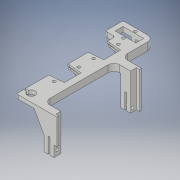
# Autodesk Inventor part: stand2
Saved by Autodesk Inventor 2019 (Build 230136000, 136)
## iProperties
Created: 2019-09-12
Part Number: stand2
Material: Generic
Document SubType Name: Modeling
Designer: James
Density: 1 g/cm^3
Appearance: Default
Author: James
Autodesk Inventor part; units mm, degrees
ref_plane "YZ Plane" through (0, 0, 0) normal (1, 0, 0) x (0, 1, 0)
ref_plane "XZ Plane" through (0, 0, 0) normal (0, 1, 0) x (-1, 0, 0)
ref_plane "XY Plane" through (0, 0, 0) normal (0, 0, 1) x (1, 0, 0)
sketch "Sketch1" plane through (0, 0, 0) normal (0, 1, 0) x (-1, 0, 0)
  line L0 (-9.5, 50) -> (-9.5, -50)
  line L1 (-9.5, -50) -> (9.5, -50)
  line L2 (9.5, 50) -> (9.5, -50)
  line L3 (-9.5, 50) -> (9.5, 50)
  line L4 (9.5, -24) -> (-3, -24)
  line L5 (-3, -24) -> (-3, -41)
  line L6 (-3, -41) -> (9.5, -41)
  line L7 (9.5, -41) -> (9.5, -24)
  circle A0 centre (3.25, -45) radius 1.5
  circle A1 centre (3.25, -20) radius 1.5
  line L8 (9.5, 16) -> (-3, 16)
  line L9 (-3, 16) -> (-3, -1)
  line L10 (-3, -1) -> (9.5, -1)
  circle A2 centre (3.25, -5) radius 1.5
  circle A3 centre (3.25, 20) radius 1.5
  arc A4 (8.4291, 42.75) -> (8.2997, 40.75) centre (4.5, 42) ccw
  line L11 (6.5529, 38) -> (0.8469, 38)
  line L12 (9.5, 42.75) -> (8.4291, 42.75)
  line L13 (8.2997, 40.75) -> (9.5, 40.75)
  point P0 (0, 0)
  point P1 (9.5, 0)
  point P2 (-9.5, 0)
  point P3 (-3, -32.5)
  point P4 (3.25, -24)
  point P5 (0, -50)
  point P6 (-3, 7.5)
  point P7 (3.25, 16)
  dimension "d3" = 17
  dimension "d4" = 12.5
  dimension "d5" = 12.5
  dimension "d6" = 12.5
  dimension "d7" = 100
  dimension "d8" = 19
  dimension "d9" = 17
  dimension "d10" = 12.5
  dimension "d11" = 12.5
  dimension "d12" = 12.5
  dimension "d13" = 40
  dimension "d14" = 3
  dimension "d15" = 17.5
  dimension "d16" = 8
  dimension "d18" = 5
  dimension "d19" = 2
  dimension "d20" = 0.75
  dimension "d68" = 8
  constraints: 28 end point, 7 midpoint, 7 perpendicular, 5 centre point, 5 point on line, 5 vertical alignment, 4 horizontal, 3 equal radius, 3 parallel, 2 horizontal alignment, 2 point on circle, 1 tangent
  measures "d3" distance of L4.end L5.end
  measures "d4" distance of L4.start L4.end
  measures "d5" vertical distance of A1.centre point (-3, -32.5)
  measures "d6" vertical distance of A0.centre point (-3, -32.5)
  measures "d7" distance of L2.start L1.end
  measures "d8" distance of L0.start L2.start
  measures "d9" distance of L8.end L9.end
  measures "d10" distance of L8.start L8.end
  measures "d11" vertical distance of A3.centre point (-3, 7.5)
  measures "d12" vertical distance of A2.centre point (-3, 7.5)
  measures "d13" distance of point (-3, -32.5) point (-3, 7.5)
  measures "d14" diameter of A3
  measures "d15" distance from line of L1 point (-3, -32.5)
  measures "d16" diameter of A4
  measures "d18" distance from line of L2 A4.centre
  measures "d19" distance between parallel lines of L13 L12
  measures "d20" vertical distance of A4.centre L12.start
  measures "d68" distance from line of L3 A4.centre
extrude "Extrusion1" add sketch "Sketch1" along normal blind 3 contours L3 L2 L12 A4 L13 L8 L9 L10 L4 L5 L6 L1 L0
sketch "Sketch2" plane through (-9.5, 0, 16) normal (-1, 0, 0) x (0, 0, 1)
  line L0 (-64.2, 0.85) -> (-64.2, 2.15)
  line L1 (7.2, 2.15) -> (7.2, 0.85)
  line L2 (-66, 0) -> (-66, 3) projected
  line L3 (-66, 3) -> (-57, 3) projected
  line L4 (-24.2, 0.85) -> (-24.2, 2.15)
  line L5 (-32.8, 0.85) -> (-32.8, 2.15)
  line L6 (-64.2, 2.15) -> (-32.8, 2.15)
  line L7 (-24.2, 2.15) -> (7.2, 2.15)
  line L8 (7.2, 0.85) -> (-24.2, 0.85)
  line L9 (-32.8, 0.85) -> (-64.2, 0.85)
  point P0 (-16, 0)
  point P1 (-24.2, 1.5)
  point P2 (-32.8, 1.5)
  point P3 (-64.2, 1.5)
  point P4 (-66, 1.5)
  dimension "d23" = 1.3
  dimension "d57" = 1.8
  dimension "d58" = 8.6
  dimension "d59" = 31.4
  dimension "d60" = 31.4
  dimension "d61" = 1.3
  constraints: 16 end point, 5 parallel, 4 midpoint, 4 perpendicular, 2 horizontal, 2 horizontal alignment
  measures "d23" distance of L1.end L1.start
  measures "d57" distance between parallel lines of L2 L0
  measures "d58" distance from line of L5 L4.end
  measures "d59" distance between parallel lines of L1 L4
  measures "d60" distance of L5.start L0.start
  measures "d61" distance of L0.start L0.end
extrude "Extrusion2" cut sketch "Sketch2" against normal blind 13
sketch "Sketch11" plane through (0, 3, 0) normal (0, 1, 0) x (1, 0, 0)
  line L0 (-9.5, -16) -> (-9.5, -40.75) projected
  line L1 (-9.5, -17.1) -> (3, -16)
  line L2 (3, -16) -> (-9.5, -16)
  line L3 (3, 1) -> (3, -16) projected
  line L4 (-9.5, -16) -> (-9.5, -17.1)
  line L5 (-9.5, 1) -> (3, 1) projected
  line L6 (-9.5, 1) -> (3, 1)
  line L7 (3, 1) -> (-9.5, 2.1)
  line L8 (-9.5, 24) -> (-9.5, 1) projected
  line L9 (-9.5, 1) -> (3, 1)
  line L10 (3, 41) -> (3, 24) projected
  line L11 (3, 24) -> (-9.5, 22.9)
  line L12 (-9.5, 24) -> (-9.5, 16.8) projected
  line L13 (-9.5, 24) -> (3, 24)
  line L14 (3.5, 48.2) -> (3.5, 41) projected
  line L15 (-9.5, 48.2) -> (-9.5, 41) projected
  line L16 (3, 41) -> (-9.5, 41)
  line L17 (3, 41) -> (-9.5, 42.1)
  line L18 (-9.5, 1) -> (-9.5, 2.1)
  line L19 (-9.5, 22.9) -> (-9.5, 24)
  line L20 (-9.5, 41) -> (-9.5, 42.1)
  point P0 (0, 0)
  dimension "d62" = 1.1
  dimension "d63" = 1.1
  dimension "d64" = 1.1
  dimension "d65" = 1.1
  constraints: 26 end point, 4 collinear, 4 point on line, 3 perpendicular, 2 horizontal
  measures "d62" distance of L2.end L1.start
  measures "d63" distance of L7.end L5.start
  measures "d64" distance of L8.start L11.end
  measures "d65" distance of L17.end L15.end
extrude "Extrusion11" cut sketch "Sketch11" against normal blind 4.75
sketch "Sketch12" plane through (0, 0, 0) normal (0, -1, 0) x (1, 0, 0)
  point P0 (0, 0)
sketch "Sketch13" plane through (9.5, 0, 50) normal (1, 0, 0) x (0, 0, -1)
  line L0 (0, 3) -> (100, 3) projected
  line L1 (0, 3) -> (7, 3)
  line L2 (7, 3) -> (7, 0)
  line L3 (7, 0) -> (0, 0)
  line L4 (0, 0) -> (0, 3)
  point P0 (50, 0)
  dimension "d69" = 7
  dimension "d70" = 3
  constraints: 8 end point, 2 parallel, 1 horizontal, 1 perpendicular
  measures "d69" distance of L2.end L3.end
  measures "d70" distance of L3.end L0.start
extrude "Extrusion12" add sketch "Sketch13" along normal blind 15
sketch "Sketch14" plane through (0, 0, 0) normal (0, -1, 0) x (1, 0, 0)
  line L0 (9.5, 43) -> (24.5, 43) projected
  line L1 (-9.5, 50) -> (24.5, 50) projected
  line L2 (24.5, 43) -> (18.5, 43)
  line L3 (18.5, 43) -> (18.5, 50)
  line L4 (18.5, 50) -> (24.5, 50)
  line L5 (24.5, 50) -> (24.5, 43)
  point P0 (0, 0)
  dimension "d73" = 6
  constraints: 8 end point, 2 parallel, 1 horizontal, 1 perpendicular, 1 point on line
  measures "d73" distance of L3.end L4.end
extrude "Extrusion13" add sketch "Sketch14" along normal blind 17
sketch "Sketch15" plane through (0, -17, 0) normal (0, -1, 0) x (1, 0, 0)
  line L0 (9.5, 43) -> (24.5, 43) projected
  line L1 (-9.5, 50) -> (24.5, 50) projected
  line L2 (18.5, 43) -> (20.5, 43)
  line L3 (20.5, 43) -> (20.5, 50)
  line L4 (20.5, 50) -> (18.5, 50)
  line L5 (18.5, 50) -> (18.5, 43)
  line L6 (24.5, 50) -> (22.5, 50)
  line L7 (22.5, 50) -> (22.5, 43)
  line L8 (22.5, 43) -> (24.5, 43)
  line L9 (24.5, 43) -> (24.5, 50)
  line L10 (18.5, 43) -> (24.5, 43) projected
  line L11 (18.5, 43) -> (20.5, 43)
  line L12 (20.5, 43) -> (20.5, 50)
  line L13 (20.5, 50) -> (18.5, 50)
  line L14 (18.5, 50) -> (18.5, 43)
  point P0 (0, 0)
  dimension "d76" = 2
  dimension "d77" = 2
  constraints: 24 end point, 6 parallel, 4 point on line, 3 horizontal, 3 perpendicular
  measures "d76" distance of L4.end L3.end
  measures "d77" distance of L8.end L7.end
extrude "Extrusion14" add sketch "Sketch15" along normal blind 16 contours L5 L1 L3 L0 | L7 L1 L9 L0
sketch "Sketch16" plane through (-9.5, 0, 50) normal (0, 0, 1) x (1, 0, 0)
  line L0 (28, 0) -> (28, -33) projected
  line L1 (28, -22) -> (16, 0)
  line L2 (19, 0) -> (0, 0) projected
  line L3 (28, -22) -> (28, 0)
  line L4 (19, 3) -> (34, 3) projected
  line L5 (0, 0) -> (28, 0) projected
  line L6 (16, 0) -> (28, 0)
  point P0 (9.5, 0)
  dimension "d80" = 12
  dimension "d81" = 22
  constraints: 6 end point, 2 point on line, 1 horizontal, 1 perpendicular
  measures "d80" distance of L0.start L1.end
  measures "d81" distance of L0.start L1.start
extrude "Extrusion15" add sketch "Sketch16" against normal blind 2
sketch "Sketch17" plane through (18.5, -33, 43) normal (-1, 0, 0) x (0, 0, 1)
  circle A0 centre (3.5, 5.13) radius 1.5
  line L0 (0, 33) -> (0, 0) projected
  point P0 (-43, 33)
  point P1 (0, 16)
  dimension "d84" = 3
  dimension "d85" = 3.5
  dimension "d86" = 10.87
  constraints: 1 centre point
  measures "d84" diameter of A0
  measures "d85" distance from line of A0.centre L0
  measures "d86" vertical distance of point (0, 16) A0.centre
extrude "Extrusion16" cut sketch "Sketch17" against normal blind 6
sketch "Sketch19" plane through (18.5, -33, 43) normal (-1, 0, 0) x (0, 0, 1)
  circle A0 centre (-72.7, 3.86) radius 1.5
  circle A1 centre (3.5, 5.13) radius 1.5 projected
  line L0 (0, 33) -> (-93, 33) projected
  line L1 (-78.7, 33) -> (-70.7, 33)
  line L2 (-70.7, 33) -> (-70.7, 0)
  line L3 (-70.7, 0) -> (-78.7, 0)
  line L4 (-78.7, 0) -> (-78.7, 33)
  line L5 (7, 0) -> (0, 0) projected
  point P0 (-43, 33)
  point P1 (-74.7, 0)
  point P2 (3.5, 0)
  dimension "d89" = 76.2
  dimension "d90" = 1.27
  dimension "d91" = 3
  dimension "d92" = 2
  dimension "d93" = 8
  constraints: 8 end point, 2 midpoint, 2 parallel, 1 centre point, 1 horizontal, 1 horizontal alignment, 1 perpendicular, 1 point on line
  measures "d89" horizontal distance of A1.centre A0.centre
  measures "d90" vertical distance of A1.centre A0.centre
  measures "d91" diameter of A0
  measures "d92" distance from line of L2 A0.centre
  measures "d93" distance between parallel lines of L2 L4
extrude "Extrusion17" add sketch "Sketch19" against normal blind 6 contours L2 L3 L4 L0
sketch "Sketch20" plane through (18.5, 0, -27.7) normal (0, 1, 0) x (1, 0, 0)
  line L0 (6, 8) -> (6, 0) projected
  line L1 (-9, -70.7) -> (-9, 22.3) projected
  line L2 (6, 0) -> (-9, 0)
  line L3 (-9, 0) -> (-9, 8)
  line L4 (-9, 8) -> (6, 8)
  line L5 (6, 8) -> (6, 0)
  point P0 (-18.5, -27.7)
  point P1 (-1.5, 8)
  constraints: 8 end point, 2 parallel, 1 horizontal, 1 horizontal alignment, 1 midpoint, 1 perpendicular, 1 point on line
extrude "Extrusion18" add sketch "Sketch20" along normal blind 3
sketch "Sketch21" plane through (18.5, -33, -35.7) normal (0, -1, 0) x (1, 0, 0)
  line L0 (6, 0) -> (-9, 0) projected
  line L1 (2, 0) -> (4, 0)
  line L2 (4, 0) -> (4, 8)
  line L3 (4, 8) -> (2, 8)
  line L4 (2, 8) -> (2, 0)
  line L5 (0, 8) -> (0, 0) projected
  point P0 (-18.5, 35.7)
  dimension "d98" = 8
  dimension "d99" = 2
  dimension "d100" = 2
  constraints: 8 end point, 2 parallel, 1 horizontal, 1 perpendicular, 1 point on line
  measures "d98" distance of L1.end L2.end
  measures "d99" distance of L2.end L3.end
  measures "d100" distance between parallel lines of L5 L4
extrude "Extrusion19" cut sketch "Sketch21" against normal blind 16
sketch "Sketch22" plane through (18.5, 0, -35.7) normal (0, 0, -1) x (-1, 0, 0)
  line L0 (28, 0) -> (12, 0) projected
  line L1 (12, 0) -> (0, -22)
  line L2 (12, 0) -> (0, 0)
  line L3 (0, 0) -> (0, -22)
  point P0 (18.5, 0)
  constraints: 6 end point, 1 horizontal, 1 perpendicular
extrude "Extrusion20" add sketch "Sketch22" against normal blind 2
fillet "Fillet2" radius 6 3 edges at (9.5, 1.5, -27.7) (9.5, 1.5, 43) (9.5, 1.5, -35.7)
sketch "Sketch23" plane through (24.5, -33, 43) normal (1, 0, 0) x (0, 0, -1)
  line L0 (78.7, 36) -> (76.7, 36)
  line L1 (76.7, 36) -> (76.7, 0)
  line L2 (76.7, 0) -> (78.7, 0)
  line L3 (78.7, 0) -> (78.7, 36)
  line L4 (-7, 36) -> (-7, 0) projected
  line L5 (-7, 36) -> (-5, 36)
  line L6 (-5, 36) -> (-5, 11)
  line L7 (-5, 11) -> (-7, 11)
  line L8 (-7, 11) -> (-7, 36)
  point P0 (43, 33)
  point P1 (77.7, 0)
  point P2 (-6, 11)
  dimension "d106" = 2
  dimension "d107" = 2
  dimension "d108" = 25
  constraints: 16 end point, 4 parallel, 2 horizontal, 2 midpoint, 2 perpendicular, 1 point on line
  measures "d106" distance of L1.end L2.end
  measures "d107" distance of L6.end L7.end
  measures "d108" distance between parallel lines of L5 L7
extrude "Extrusion21" add sketch "Sketch23" along normal blind 5
sketch "Sketch24" plane through (0, 0, 0) normal (0, -1, 0) x (1, 0, 0)
  circle A0 centre (-3.25, -45) radius 1.5
  circle A1 centre (-3.25, -45) radius 3
  circle A2 centre (-3.25, -20) radius 1.5
  circle A3 centre (-3.25, -20) radius 1.5
  circle A4 centre (-3.25, -20) radius 3
  circle A5 centre (-3.25, -5) radius 1.5
  circle A6 centre (-3.25, -5) radius 3
  circle A7 centre (-3.25, 20) radius 1.5
  circle A8 centre (-3.25, 20) radius 3
  circle A9 centre (-3.25, -45) radius 1.5 projected
  circle A10 centre (-3.25, -20) radius 1.5 projected
  circle A11 centre (-3.25, -5) radius 1.5 projected
  circle A12 centre (-3.25, 20) radius 1.5 projected
  point P0 (0, 0)
  dimension "d113" = 6
  constraints: 9 centre point, 8 equal radius, 5 coincident, 4 concentric
  measures "d113" diameter of A1
extrude "Extrusion22" add sketch "Sketch24" along normal blind 2
sketch "Sketch25" plane through (0, 0, 0) normal (0, -1, 0) x (1, 0, 0)
  line L0 (-9.5, -42.1) -> (3, -41) projected
  line L1 (3, -41) -> (-9.5, -42.929)
  line L2 (-9.5, -50) -> (-9.5, -42.1) projected
  line L3 (3, -41) -> (3, -24) projected
  line L4 (3, -41) -> (-9.5, -42.1)
  line L5 (-9.5, -42.1) -> (-9.5, -42.929)
  line L6 (-9.5, -50) -> (-9.5, -42.1) projected
  circle A0 centre (-3.25, -45) radius 3 projected
  line L7 (-9.5, -22.9) -> (-9.5, -2.1) projected
  line L8 (3, -24) -> (-9.5, -22.9)
  line L9 (-9.5, -16.8) -> (-9.5, -22.9) projected
  line L10 (-9.5, -22.9) -> (-9.5, -22.071)
  line L11 (-9.5, -22.071) -> (3, -24)
  circle A1 centre (-3.25, -20) radius 3 projected
  line L12 (3, -1) -> (3, 16) projected
  line L13 (3, -1) -> (-9.5, -2.929)
  line L14 (-9.5, -2.1) -> (-9.5, -8.2) projected
  line L15 (-9.5, -2.1) -> (-9.5, -2.929)
  line L16 (3, -1) -> (-9.5, -2.1) projected
  line L17 (-9.5, -2.1) -> (3, -1)
  circle A2 centre (-3.25, -5) radius 3 projected
  line L18 (3.5, 23.2) -> (3.5, 16) projected
  line L19 (-9.5, 17.1) -> (3, 16) projected
  line L20 (3, 16) -> (-9.5, 17.1)
  line L21 (-9.5, 17.1) -> (-9.5, 17.929)
  line L22 (-9.5, 17.1) -> (-9.5, 40.75) projected
  line L23 (3, 16) -> (-9.5, 17.929)
  circle A3 centre (-3.25, 20) radius 3 projected
  point P0 (0, 0)
  constraints: 24 end point, 5 collinear, 4 point on line, 4 tangent
extrude "Extrusion23" cut sketch "Sketch25" against normal blind 1 contours L0 L1 L2 | L7 L11 L8 | L7 L16 L13 | L21 L23 L19
sketch "Sketch26" plane through (0, 0, 0) normal (0, -1, 0) x (1, 0, 0)
  arc A0 (9.5, -21.7) -> (15.5, -27.7) centre (15.5, -21.7) ccw
  arc A1 (9.5, -21.7) -> (15.5, -27.7) centre (15.5, -21.7) ccw projected
  arc A2 (15.5, 43) -> (9.5, 37) centre (15.5, 37) ccw projected
  line L0 (9.5, 37) -> (9.5, -21.7) projected
  line L1 (9.5, 37) -> (9.5, -21.7) projected
  line L2 (9.5, -21.7) -> (9.5, 37)
  line L3 (18.5, -27.7) -> (18.5, -35.7) projected
  arc A3 (9.5, -21.7) -> (15.5, -27.7) centre (15.5, -21.7) ccw projected
  line L4 (18.5, -27.7) -> (15.5, -27.7)
  arc A4 (7.5, -21.7) -> (15.5, -29.7) centre (15.5, -21.7) ccw
  line L5 (18.5, -31.2) -> (18.5, -28.2) projected
  line L6 (18.5, -29.7) -> (15.5, -29.7)
  arc A5 (15.5, 45) -> (7.5, 37) centre (15.5, 37) ccw
  line L7 (7.5, -21.7) -> (7.5, 37)
  line L8 (15.5, 45) -> (18.5, 45)
  line L9 (18.5, 43) -> (18.5, 48) projected
  line L10 (18.5, 50) -> (18.5, 43) projected
  arc A6 (15.5, 43) -> (9.5, 37) centre (15.5, 37) ccw
  line L11 (15.5, 43) -> (18.5, 43) projected
  line L12 (18.5, 43) -> (15.5, 43)
  point P0 (0, 0)
  dimension "d118" = 16
  dimension "d119" = 16
  constraints: 13 end point, 9 tangent, 8 point on circle, 4 centre point, 3 coincident, 3 equal length, 3 perpendicular, 2 concentric, 1 horizontal, 1 midpoint, 1 point on line
  measures "d118" diameter of A4
  measures "d119" diameter of A5
extrude "Extrusion24" add sketch "Sketch26" along normal blind 3
sketch "Sketch27" plane through (0, 3, 0) normal (0, 1, 0) x (1, 0, 0)
  line L0 (9.5, 50) -> (-9.5, 50) projected
  line L1 (-9.5, 50) -> (-9.5, 42.1) projected
  line L2 (-9.5, 42.1) -> (3, 41) projected
  line L3 (3, 41) -> (3, 24) projected
  line L4 (3, 24) -> (-9.5, 22.9) projected
  line L5 (-9.5, 22.9) -> (-9.5, 2.1) projected
  line L6 (-9.5, 2.1) -> (3, 1) projected
  line L7 (3, 1) -> (3, -16) projected
  line L8 (3, -16) -> (-9.5, -17.1) projected
  line L9 (-9.5, -17.1) -> (-9.5, -40.75) projected
  line L10 (-9.5, -40.75) -> (-8.2997, -40.75) projected
  arc A0 (-8.4291, -42.75) -> (-8.2997, -40.75) centre (-4.5, -42) ccw projected
  line L11 (-8.4291, -42.75) -> (-9.5, -42.75) projected
  line L12 (-9.5, -42.75) -> (-9.5, -50) projected
  line L13 (-9.5, -50) -> (29.5, -50) projected
  line L14 (29.5, -48) -> (29.5, -50) projected
  line L15 (24.5, -48) -> (29.5, -48) projected
  line L16 (24.5, -43) -> (24.5, -48) projected
  line L17 (15.5, -43) -> (24.5, -43) projected
  arc A1 (9.5, -37) -> (15.5, -43) centre (15.5, -37) ccw projected
  line L18 (9.5, -37) -> (9.5, 21.7) projected
  arc A2 (15.5, 27.7) -> (9.5, 21.7) centre (15.5, 21.7) ccw projected
  line L19 (15.5, 27.7) -> (24.5, 27.7) projected
  line L20 (24.5, 27.7) -> (24.5, 33.7) projected
  line L21 (24.5, 33.7) -> (29.5, 33.7) projected
  line L22 (29.5, 35.7) -> (29.5, 33.7) projected
  line L23 (15.5, 35.7) -> (29.5, 35.7) projected
  arc A3 (9.5, 41.7) -> (15.5, 35.7) centre (15.5, 41.7) ccw projected
  line L24 (9.5, 41.7) -> (9.5, 50) projected
  circle A4 centre (-3.25, -20) radius 1.5 projected
  circle A5 centre (-3.25, 5) radius 1.5 projected
  circle A6 centre (-3.25, 20) radius 1.5 projected
  circle A7 centre (-3.25, 45) radius 1.5 projected
  point P0 (0, 0)
extrude "Extrusion25" add sketch "Sketch27" along normal blind 1
sketch "Sketch28" plane through (24.5, 0, 50) normal (1, 0, 0) x (0, 0, -1)
  line L0 (83.7, -33) -> (83.7, 4) projected
  line L1 (77.7, 4) -> (83.7, 4) projected
  line L2 (77.7, -33) -> (77.7, 4) projected
  line L3 (77.7, -33) -> (83.7, -33) projected
  circle A0 centre (79.7, -29.14) radius 1.5 projected
  line L4 (2, -22) -> (0, -22) projected
  line L5 (0, -22) -> (0, -33) projected
  line L6 (7, -33) -> (0, -33) projected
  line L7 (7, 4) -> (7, -33) projected
  line L8 (2, 4) -> (7, 4) projected
  line L9 (2, 4) -> (2, -22) projected
  circle A1 centre (3.5, -27.87) radius 1.5 projected
  point P0 (50, 0)
extrude "Extrusion26" add sketch "Sketch28" along normal blind 2
sketch "Sketch29" plane through (18.5, -33, 43) normal (-1, 0, 0) x (0, 0, 1)
  line L0 (2, 33) -> (2, 30) projected
  line L1 (2, 30) -> (0, 30) projected
  line L2 (0, 30) -> (0, 0) projected
  line L3 (7, 0) -> (0, 0) projected
  line L4 (7, 11) -> (7, 0) projected
  line L5 (7, 11) -> (5, 11) projected
  line L6 (5, 11) -> (5, 33) projected
  line L7 (2, 33) -> (5, 33) projected
  circle A0 centre (3.5, 5.13) radius 1.5 projected
  line L8 (-72.7, 30) -> (-72.7, 33) projected
  line L9 (-76.7, 33) -> (-72.7, 33) projected
  line L10 (-76.7, 33) -> (-76.7, 11) projected
  line L11 (-76.7, 11) -> (-78.7, 11) projected
  line L12 (-78.7, 0) -> (-78.7, 11) projected
  line L13 (-70.7, 0) -> (-78.7, 0) projected
  line L14 (-70.7, 30) -> (-70.7, 0) projected
  line L15 (-70.7, 30) -> (-72.7, 30) projected
  circle A1 centre (-72.7, 3.86) radius 1.5 projected
  point P0 (-43, 33)
extrude "Extrusion27" add sketch "Sketch29" along normal blind 2
sketch "Sketch30" plane through (18.5, -22, -33.7) normal (0, 0, -1) x (-1, 0, 0)
  line L0 (2, 3.6667) -> (0, 0) projected
  line L1 (0, 0) -> (2, 0) projected
  line L2 (2, 3.6667) -> (2, 0) projected
  point P0 (18.5, 22)
extrude "Extrusion28" add sketch "Sketch30" along normal blind 2
sketch "Sketch31" plane through (16.5, -22, 48) normal (0, 0, 1) x (1, 0, 0)
  line L0 (2, 0) -> (0, 3.6667) projected
  line L1 (0, 0) -> (0, 3.6667) projected
  line L2 (2, 0) -> (0, 0) projected
  point P0 (-16.5, 22)
extrude "Extrusion29" add sketch "Sketch31" along normal blind 2
sketch "Sketch32" plane through (0, 0, 0) normal (0, -1, 0) x (1, 0, 0)
  line L0 (16.5, 45) -> (16.5, 48) projected
  line L1 (16.5, 48) -> (6.5, 48) projected
  line L2 (6.5, 48) -> (6.5, 50) projected
  line L3 (-9.5, 50) -> (6.5, 50) projected
  line L4 (-9.5, 42.75) -> (-9.5, 50) projected
  line L5 (-8.4291, 42.75) -> (-9.5, 42.75) projected
  arc A0 (-8.2997, 40.75) -> (-8.4291, 42.75) centre (-4.5, 42) ccw projected
  line L6 (-9.5, 40.75) -> (-8.2997, 40.75) projected
  line L7 (-9.5, 17.929) -> (-9.5, 40.75) projected
  line L8 (-9.5, 17.929) -> (-3.7075, 17.0351) projected
  circle A1 centre (-3.25, 20) radius 3 projected
  line L9 (-3.7075, 17.0351) -> (3, 16) projected
  line L10 (3, -1) -> (3, 16) projected
  line L11 (3, -1) -> (-3.7075, -2.0351) projected
  circle A2 centre (-3.25, -5) radius 3 projected
  line L12 (-3.7075, -2.0351) -> (-9.5, -2.929) projected
  line L13 (-9.5, -22.071) -> (-9.5, -2.929) projected
  line L14 (-9.5, -22.071) -> (-3.7075, -22.9649) projected
  circle A3 centre (-3.25, -20) radius 3 projected
  line L15 (-3.7075, -22.9649) -> (3, -24) projected
  line L16 (3, -24) -> (3, -41) projected
  line L17 (3, -41) -> (-3.7075, -42.0351) projected
  circle A4 centre (-3.25, -45) radius 3 projected
  line L18 (-3.7075, -42.0351) -> (-9.5, -42.929) projected
  line L19 (-9.5, -50) -> (-9.5, -42.929) projected
  line L20 (9.5, -50) -> (-9.5, -50) projected
  line L21 (9.5, -41.7) -> (9.5, -50) projected
  arc A5 (15.5, -35.7) -> (9.5, -41.7) centre (15.5, -41.7) ccw projected
  line L22 (15.5, -35.7) -> (6.5, -35.7) projected
  line L23 (6.5, -35.7) -> (6.5, -33.7) projected
  line L24 (6.5, -33.7) -> (16.5, -33.7) projected
  line L25 (16.5, -33.7) -> (16.5, -29.7) projected
  line L26 (16.5, -29.7) -> (15.5, -29.7) projected
  arc A6 (7.5, -21.7) -> (15.5, -29.7) centre (15.5, -21.7) ccw projected
  line L27 (7.5, -21.7) -> (7.5, 37) projected
  arc A7 (15.5, 45) -> (7.5, 37) centre (15.5, 37) ccw projected
  line L28 (15.5, 45) -> (16.5, 45) projected
  line L29 (-9.5, 17.929) -> (-9.5, 40.75) projected
  line L30 (-9.5, 29.3395) -> (7.5, 29.3395)
  point P0 (0, 0)
  constraints: 2 end point, 1 horizontal, 1 midpoint, 1 point on line, 4 other
extrude "Extrusion30" add sketch "Sketch32" along normal blind 1 contours L27 A6 L26 L25 L24 L23 L22 A5 L21 L20 L19 L18 L17 L16 L15 L14 L13 L12 L11 L10 L9 L8 L7 L30
sketch "Sketch33" plane through (7.0455, -1, -33.7) normal (0, 0, -1) x (-1, 0, 0)
  line L0 (0.5455, 1) -> (0, 0) projected
  line L1 (0.5455, 0) -> (0, 0) projected
  line L2 (0.5455, 1) -> (0.5455, 0) projected
  point P0 (7.0455, 1)
extrude "Extrusion31" add sketch "Sketch33" along normal blind 2
sketch "Sketch34" plane through (-9.5, 0.85, -8.2) normal (-1, 0, 0) x (0, 0, 1)
  line L0 (-34.729, -1.85) -> (-34.729, 0) projected
  line L1 (-34.729, 0) -> (-40, 0) projected
  line L2 (-40, 0) -> (-40, 1.3) projected
  line L3 (-40, 1.3) -> (-33.9, 1.3) projected
  line L4 (-33.9, 1.3) -> (-33.9, 3.15) projected
  line L5 (-41.8, 3.15) -> (-33.9, 3.15) projected
  line L6 (-41.8, -1.85) -> (-41.8, 3.15) projected
  line L7 (-34.729, -1.85) -> (-41.8, -1.85) projected
  line L8 (-13.871, 0) -> (-13.871, -1.85) projected
  line L9 (5.271, -1.85) -> (-13.871, -1.85) projected
  line L10 (5.271, -1.85) -> (5.271, 0) projected
  line L11 (5.271, 0) -> (0, 0) projected
  line L12 (0, 0) -> (0, 1.3) projected
  line L13 (0, 1.3) -> (6.1, 1.3) projected
  line L14 (6.1, 1.3) -> (6.1, 3.15) projected
  line L15 (-14.7, 3.15) -> (6.1, 3.15) projected
  line L16 (-14.7, 3.15) -> (-14.7, 1.3) projected
  line L17 (-14.7, 1.3) -> (-8.6, 1.3) projected
  line L18 (-8.6, 1.3) -> (-8.6, 0) projected
  line L19 (-8.6, 0) -> (-13.871, 0) projected
  line L20 (26.129, 0) -> (26.129, -1.85) projected
  line L21 (37.5395, -1.85) -> (26.129, -1.85) projected
  line L22 (37.5395, -0.85) -> (37.5395, -1.85) projected
  line L23 (37.5395, -0.85) -> (48.95, -0.85) projected
  line L24 (48.95, -0.85) -> (48.95, 3.15) projected
  line L25 (25.3, 3.15) -> (48.95, 3.15) projected
  line L26 (25.3, 3.15) -> (25.3, 1.3) projected
  line L27 (25.3, 1.3) -> (31.4, 1.3) projected
  line L28 (31.4, 1.3) -> (31.4, 0) projected
  line L29 (31.4, 0) -> (26.129, 0) projected
  line L30 (50.95, -0.85) -> (58.2, -0.85) projected
  line L31 (58.2, -0.85) -> (58.2, 3.15) projected
  line L32 (50.95, 3.15) -> (58.2, 3.15) projected
  line L33 (50.95, -0.85) -> (50.95, 3.15) projected
  point P0 (8.2, -0.85)
extrude "Extrusion32" add sketch "Sketch34" along normal blind 2
sketch "Sketch35" plane through (0, -1, 0) normal (0, -1, 0) x (1, 0, 0)
  line L0 (9.5, -50) -> (9.5, -41.7) projected
  line L1 (9.5, -50) -> (-21.5, -50)
  line L2 (-21.5, -50) -> (-21.5, -68)
  line L3 (-21.5, -68) -> (9.5, -68)
  line L4 (9.5, -68) -> (9.5, -50)
  line L5 (4.5, -55) -> (-16.5, -55)
  line L6 (-16.5, -55) -> (-16.5, -63)
  line L7 (-16.5, -63) -> (4.5, -63)
  line L8 (4.5, -63) -> (4.5, -55)
  point P0 (0, 0)
  dimension "d138" = 5
  dimension "d139" = 5
  dimension "d140" = 5
  dimension "d141" = 5
  dimension "d142" = 21
  dimension "d143" = 8
  constraints: 16 end point, 4 parallel, 2 horizontal, 2 perpendicular
  measures "d138" distance between parallel lines of L1 L5
  measures "d139" distance between parallel lines of L2 L6
  measures "d140" distance between parallel lines of L4 L8
  measures "d141" distance between parallel lines of L3 L7
  measures "d142" distance of L6.end L7.end
  measures "d143" distance of L5.end L6.end
extrude "Extrusion33" add sketch "Sketch35" against normal blind 5
sketch "Sketch36" plane through (0, -1, 0) normal (0, -1, 0) x (1, 0, 0)
  arc A0 (-8.2361, -63) -> (-3.7639, -63) centre (-6, -65) ccw
  arc A1 (-3.7639, -55) -> (-8.2361, -55) centre (-6, -53) ccw
  circle A2 centre (-6, -65) radius 1.5
  circle A3 centre (-6, -53) radius 1.5
  line L0 (-16.5, -55) -> (4.5, -55) projected
  line L1 (4.5, -63) -> (-16.5, -63) projected
  point P0 (0, 0)
  point P1 (-6, -55)
  dimension "d146" = 6
  dimension "d147" = 3
  dimension "d148" = 2
  dimension "d149" = 2
  constraints: 4 centre point, 4 point on circle, 4 point on line, 2 coincident, 2 equal radius, 2 vertical alignment, 1 midpoint
  measures "d146" diameter of A0
  measures "d147" diameter of A2
  measures "d148" distance from line of L1 A0.centre
  measures "d149" distance from line of L0 A1.centre
extrude "Extrusion34" add sketch "Sketch36" along normal blind 4
sketch "Sketch37" plane through (0, -5, 0) normal (0, -1, 0) x (1, 0, 0)
  circle A0 centre (-6, -65) radius 1.5 projected
  circle A1 centre (-6, -53) radius 1.5 projected
  point P0 (0, 0)
extrude "Extrusion35" cut sketch "Sketch37" against normal blind 40
fillet "Fillet4" radius 2 4 edges at (-21.5, 1.5, -68) (-21.5, 1.5, -50) (-11.5, 1.5, -50) (-11.5, 2, 50)
fillet "Fillet5" radius 6 1 edges at (9.5, 1.5, -68)
sketch "Sketch38" plane through (0, -1, 0) normal (0, -1, 0) x (1, 0, 0)
  arc A0 (3.5, -68) -> (9.5, -62) centre (3.5, -62) ccw projected
  line L0 (9.5, -62) -> (9.5, -41.7) projected
  arc A1 (15.5, -35.7) -> (9.5, -41.7) centre (15.5, -41.7) ccw projected
  line L1 (-6, -68) -> (3.5, -68) projected
  arc A2 (-8.2361, -63) -> (-3.7639, -63) centre (-6, -65) ccw projected
  arc A3 (3.5, -66) -> (7.5, -62) centre (3.5, -62) ccw
  arc A4 (10.2085, -35.7) -> (7.5, -41.7) centre (15.5, -41.7) ccw
  line L2 (7.5, -62) -> (7.5, -41.7)
  line L3 (3.5, -66) -> (-3.1716, -66)
  arc A5 (-6, -68) -> (-3.7639, -63) centre (-6, -65) ccw projected
  line L4 (7.0455, -35.7) -> (15.5, -35.7) projected
  line L5 (10.2085, -35.7) -> (15.5, -35.7)
  point P0 (0, 0)
  dimension "d156" = 2
  dimension "d157" = 2
  constraints: 6 end point, 5 point on circle, 4 tangent, 2 centre point, 2 coincident, 1 collinear, 1 parallel, 1 point on line
  measures "d156" radial gap between concentric circles of A0 A3
  measures "d157" radial gap between concentric circles of A1 A4
extrude "Extrusion36" add sketch "Sketch38" along normal blind 3
body "Solid1"
